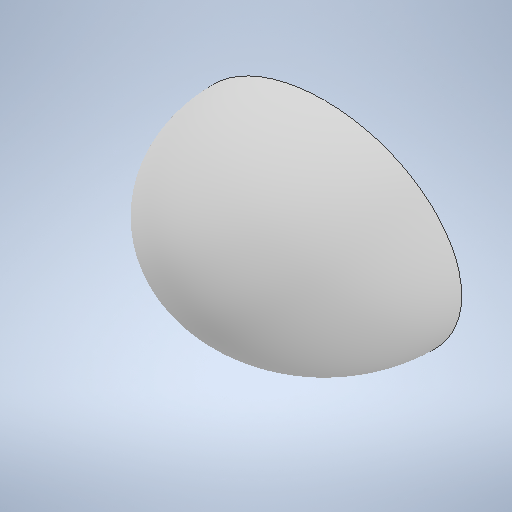
# Autodesk Inventor part: Belly
Saved by Autodesk Inventor 2025 (Build 290162000, 162)
## iProperties
Created: 2024-05-08
Part Number: Belly
Material: Generic
Document SubType Name: Modeling
Designer: Frederik Thrane
Density: 1 g/cm^3
Appearance: Default
Author: Frederik Thrane
Autodesk Inventor part; units mm, degrees
ref_plane "YZ Plane" through (0, 0, 0) normal (1, 0, 0) x (0, 1, 0)
ref_plane "XZ Plane" through (0, 0, 0) normal (0, 1, 0) x (-1, 0, 0)
ref_plane "XY Plane" through (0, 0, 0) normal (0, 0, 1) x (1, 0, 0)
sketch "Sketch6" plane through (0, 0, 0) normal (0, 0, 1) x (1, 0, 0)
  ellipse E0 centre (0, 0) end of major axis (0, 220) minor radius 300
  line L0 (0, 220) -> (0, -220)
  constraints: 2 end point, 1 vertical, 4 other
revolve "Revolution1" add sketch "Sketch6" angle 180 about axis through (0, 220, 0) along (0, -1, 0) picked at (53.9571, 71.7283) contours L0 E0
body "Solid1"
